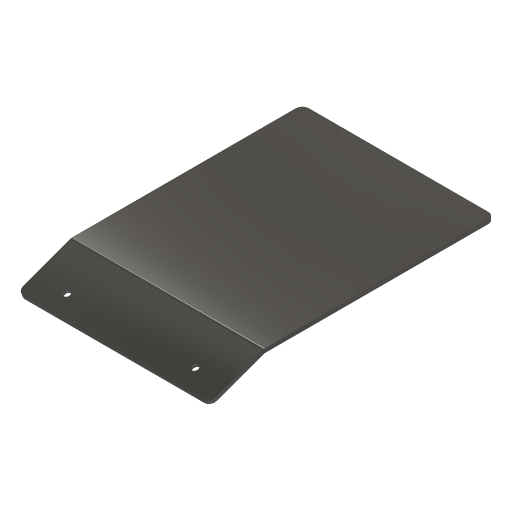
# Autodesk Inventor part: fin
Saved by Autodesk Inventor 2024.3 (Build 283343000, 343)
## iProperties
Category: 10
RuleStatus: InUse
Created: 2025-04-28
Part Number: fin
Material: S235JR(1.0038)
Description: BL3,0 0x0
Document SubType Name: Konstrukcja blachowa
Designer: Paweł Mikołaj
Mass: 576.978 g
Surface Area: 509.102 cm^2
Volume: 73.5004 cm^3
Density: 7.85 g/cm^3
Sheet Metal Rule: Default_mm
Sheet Metal Width: 0,000 mm
Sheet Metal Length: 0,000 mm
Sheet Metal Area: 0,000 mm^2
Appearance: Steel - Polished
BeforeDocSave0: file://blacha_iprop_template
Grubosc: 3,000 mm
length: =<Sheet Metal Length>
width: =<Sheet Metal Width>
Author: Paweł Mikołaj
Revision Number: 00
Autodesk Inventor part; units mm, degrees
ref_plane "YZ Plane" through (0, 0, 0) normal (1, 0, 0) x (0, 1, 0)
ref_plane "XZ Plane" through (0, 0, 0) normal (0, 1, 0) x (-1, 0, 0)
ref_plane "XY Plane" through (0, 0, 0) normal (0, 0, 1) x (1, 0, 0)
sketch "Sketch3" plane through (0, 0, 0) normal (0, 0, 1) x (1, 0, 0)
  line L0 (-75, -90) -> (75, -90)
  line L1 (75, -90) -> (75, 90)
  line L2 (75, 90) -> (-75, 90)
  line L3 (-75, 90) -> (-75, -90)
  line L4 (-75, -90) -> (75, 90) construction
  line L5 (75, -90) -> (-75, 90) construction
  point P0 (0, 0)
  dimension "d11" = 150
  dimension "d12" = 180
  measures "d11" distance of L2.end L1.end
  measures "d12" distance of L1.end L0.end
extrude "Plate3" add sketch "Sketch3" along normal blind 3
sketch "Sketch4" plane through (-75, -88.9739, 0.1809) normal (0, -0.3420201, 0.9396926) x (1, 0, 0)
  line L0 (150, 0) -> (0, 0)
  line L1 (0, 0) -> (0, -45)
  line L2 (0, -45) -> (150, -45)
  line L3 (150, -45) -> (150, 0)
  constraints: 6 end point, 1 horizontal, 1 perpendicular, 1 vertical
edge flange "Flange2" height 45 angle 20 thickness 3 bend radius 3 thickness toward (0, -0.3420201, 0.9396926) relief tear relief width 3 relief depth 1.5 edges at (0, -90, 0) wall of the first edge with corners at (75, -88.9739, 0.1809) (-75, -88.9739, 0.1809) (-75, -131.2601, -15.21) (75, -131.2601, -15.21)
bend "Bend2"
corner "Corner2"
fillet "Fillet1" radius 5 4 edges at (75, 90, 1.5) (-75, 90, 1.5) (-75, -131.7731, -13.8004) (75, -131.7731, -13.8004)
sketch "Sketch6" plane through (0, 0, 3) normal (0, 0, 1) x (1, 0, 0)
  line L0 (-67.272, 87) -> (67.272, 87) construction
  line L1 (67.272, 87) -> (67.272, -48) construction
  line L2 (67.272, -48) -> (-67.272, -48) construction
  line L3 (-67.272, -48) -> (-67.272, 87) construction
  line L4 (-75, -88.942) -> (75, -88.942) projected
  line L5 (-70, 90) -> (70, 90) projected
  point P0 (0, 0)
  point P1 (0, 87)
  point P2 (0, 90)
  dimension "d50" = 178.942
  dimension "d51" = 140
  dimension "d52" = 135
  dimension "d53" = 3
  constraints: 2 midpoint, 1 vertical alignment, 2 other
  measures "d50" distance between parallel lines of L4 L5
  measures "d51" distance of L5.start L5.end
  measures "d52" distance of L0.end L1.end
  measures "d53" distance between parallel lines of L5 L0
decal "Decal2"
sketch "Sketch7" plane through (-75, -90.9942, 2.6382) normal (0, -0.3420201, 0.9396926) x (1, 0, 0)
  line L0 (150, 0) -> (150, -38.942) projected
  line L1 (0, -38.942) -> (0, 0) projected
  line L2 (145, -43.942) -> (5, -43.942) projected
  point P0 (75, 84.6042)
  point P1 (25, -29.442)
  point P2 (125, -29.442)
  dimension "d62" = 100
  dimension "d63" = 150
  dimension "d64" = 25
  dimension "d65" = 14.5
  constraints: 1 horizontal alignment
  measures "d62" distance of point (125, -29.442) point (25, -29.442)
  measures "d63" distance between parallel lines of L0 L1
  measures "d64" distance from line of L0 point (125, -29.442)
  measures "d65" distance from line of L2 point (125, -29.442)
hole "Hole1" at (-50, -118.6606, -7.4316) at (50, -118.6606, -7.4316) direction (0, 0.3420201, -0.9396926) diameter 5.5 end through all clearance for "Countersunk Flat Head Screw DIN EN ISO 2009" size "M5" standard "DIN"
equation "\"d71\" = Grubosc"
equation "\"d13\" = Grubosc"
equation "\"d14\" = SzerokośćGięciaPodcięcia"
equation "\"d15\" = GłębokośćGięciaPodcięcia"
equation "\"d16\" = MinimalnaPozostałość"
equation "\"d17\" = PromieńPrzejścia"
equation "\"d20\" = PromieńGięcia"
equation "\"d21\" = RozmiarPodcięciaNarożnika"
equation "\"d22\" = Wielk_odstępu"
equation "\"d23\" = Rozmiar_promienia_Jacobiego"
equation "\"PromieńGięcia\" = Grubosc"
equation "\"SzerokośćGięciaPodcięcia\" = Grubosc"
equation "\"GłębokośćGięciaPodcięcia\" = 0.5 * Grubosc"
equation "\"RozmiarPodcięciaNarożnika\" = 4 * Grubosc"
equation "\"MinimalnaPozostałość\" = 2 * Grubosc"
equation "\"PromieńPrzejścia\" = PromieńGięcia"
equation "\"Rozmiar_promienia_Jacobiego\" = PromieńGięcia"
equation "\"Wielk_odstępu\" = Grubosc"
equation "\"Grubosc\" = 3"
body "Solid2"
